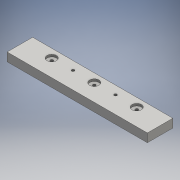
# Autodesk Inventor part: zStage_jackAttach
Saved by Autodesk Inventor 2016 (Build 200138000, 138)
## iProperties
Created: 2016-04-07
Part Number: zStage_jackAttach
Material: Generic
Document SubType Name: Modeling
Designer: sims01
Density: 1 g/cm^3
Appearance: Default
Author: sims01
Autodesk Inventor part; units mm, degrees
ref_plane "YZ Plane" through (0, 0, 0) normal (1, 0, 0) x (0, 1, 0)
ref_plane "XZ Plane" through (0, 0, 0) normal (0, 1, 0) x (-1, 0, 0)
ref_plane "XY Plane" through (0, 0, 0) normal (0, 0, 1) x (1, 0, 0)
sketch "Sketch1" plane through (0, 0, 0) normal (0, 0, 1) x (1, 0, 0)
  line L0 (-82.5, 15) -> (82.5, 15)
  line L1 (82.5, 15) -> (82.5, -15)
  line L2 (82.5, -15) -> (-82.5, -15)
  line L3 (-82.5, -15) -> (-82.5, 15)
  point P0 (0, 0)
  dimension "d0" = 165
  dimension "d1" = 30
  dimension "d2" = 82.5
  dimension "d3" = 15
  constraints: 8 end point, 2 parallel, 1 horizontal, 1 perpendicular
  measures "d0" distance of L0.start L0.end
  measures "d1" distance of L2.end L0.start
  measures "d2" distance from line of point (0, 0) L1
  measures "d3" distance from line of point (0, 0) L0
extrude "Extrusion1" add sketch "Sketch1" along normal blind 10
sketch "Sketch2" plane through (0, 0, 10) normal (0, 0, 1) x (1, 0, 0)
  line L0 (82.5, 15) -> (-82.5, 15) projected
  point P0 (0, 0)
  point P1 (-50, 5)
  point P2 (0, 5)
  point P3 (50, 5)
  dimension "d6" = 50
  dimension "d24" = 50
  dimension "d25" = 10
  constraints: 2 horizontal alignment, 1 vertical alignment
  measures "d6" distance of point (0, 5) point (-50, 5)
  measures "d24" distance of point (50, 5) point (0, 5)
  measures "d25" distance from line of point (-50, 5) L0
hole "Hole1" at (-50, 5, 10) at (0, 5, 10) at (50, 5, 10) direction (0, 0, -1) diameter 3.4 end through all counterbore diameter 11 counterbore depth 2.6 clearance for "Hex Head Cap Screw ISO 24017" size "M3" standard "ISO"
sketch "Sketch3" plane through (0, 0, 10) normal (0, 0, 1) x (1, 0, 0)
  line L0 (82.5, 15) -> (-82.5, 15) projected
  circle A0 centre (0, 5) radius 1.7 projected
  point P0 (0, 0)
  point P1 (-25, 5)
  point P2 (25, 5)
  dimension "d15" = 50
  dimension "d26" = 10
  dimension "d27" = 25
  constraints: 1 horizontal alignment
  measures "d15" distance of point (25, 5) point (-25, 5)
  measures "d26" distance from line of point (-25, 5) L0
  measures "d27" distance of A0.centre point (25, 5)
hole "Hole2" at (-25, 5, 10) at (25, 5, 10) direction (0, 0, -1) diameter 3.242 depth 11.8 tip angle 118 thread size "M4x0.7" class "6H" standard "ISO Metric profile"
equation "\"d2\" = 0.5 * d0"
equation "\"d3\" = 0.5 * d1"
equation "\"d27\" = 0.5 * d15"
body "Solid1"
